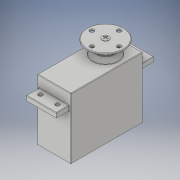
# Autodesk Inventor part: двигатель
Saved by Autodesk Inventor 2019 (Build 230136000, 136)
## iProperties
Created: 2019-09-05
Part Number: двигатель
Material: Типовые
Document SubType Name: Modeling
Designer: Iliga
Density: 1 g/cm^3
Appearance: По умолчанию
Author: Iliga
Autodesk Inventor part; units mm, degrees
sketch "Эскиз1" plane through (0, 0, 0) normal (0, 1, 0) x (-1, 0, 0)
  line L0 (-9.9, 21.15) -> (9.9, 21.15)
  line L1 (9.9, 21.15) -> (9.9, -21.15)
  line L2 (9.9, -21.15) -> (-9.9, -21.15)
  line L3 (-9.9, -21.15) -> (-9.9, 21.15)
  line L4 (-9.9, 21.15) -> (9.9, -21.15) construction
  line L5 (9.9, 21.15) -> (-9.9, -21.15) construction
  point P0 (0, 0)
  dimension "d0" = 19.8
  dimension "d1" = 42.3
  constraints: 12 end point, 2 midpoint, 2 parallel, 1 horizontal, 1 perpendicular
  measures "d0" distance of L1.end L2.end
  measures "d1" distance of L0.end L1.end
extrude "Выдавливание1" add sketch "Эскиз1" along normal blind 36.1
ref_plane "РабПлоскость1" through (0, 26.6, 0) normal (0, -1, 0) x (1, 0, 0)
sketch "Эскиз2" plane through (0, 26.6, 0) normal (0, -1, 0) x (1, 0, 0)
  line L0 (9.9, 21.15) -> (-9.9, 21.15) projected
  line L1 (-8.9, 28.75) -> (8.9, 28.75)
  line L2 (-9.9, -21.15) -> (9.9, -21.15) projected
  line L3 (-8.9, -28.75) -> (8.9, -28.75)
  line L4 (0, 28.75) -> (0, -28.75) construction
  line L5 (-9.9, 21.15) -> (9.9, 21.15)
  line L6 (9.9, -21.15) -> (9.9, 21.15) construction
  line L7 (-9.9, -21.15) -> (9.9, -21.15)
  line L8 (-8.9, 28.75) -> (-8.9, 21.15)
  line L9 (8.9, 28.75) -> (8.9, 21.15)
  line L10 (-8.9, -21.15) -> (-8.9, -28.75)
  line L11 (8.9, -21.15) -> (8.9, -28.75)
  line L12 (-9.9, 21.15) -> (-9.9, -21.15) projected
  point P0 (0, 0)
  point P1 (0, 0)
  dimension "d5" = 57.5
  dimension "d8" = 1
  constraints: 18 end point, 6 point on line, 4 perpendicular, 3 midpoint, 2 horizontal, 1 coincident, 1 collinear
  measures "d5" distance between parallel lines of L1 L3
  measures "d8" distance between parallel lines of L12 L10
extrude "Выдавливание2" add sketch "Эскиз2" against normal blind 3
sketch "Эскиз3" plane through (0, 36.1, 0) normal (0, 1, 0) x (1, 0, 0)
  circle A0 centre (0, 9.15) radius 7.5
  line L0 (9.9, 21.15) -> (-9.9, 21.15) construction
  line L1 (-9.9, 16.65) -> (9.9, 16.65) construction
  line L2 (-9.9, 21.15) -> (-9.9, -21.15) construction
  point P0 (0, 0)
  dimension "d9" = 15
  dimension "d53" = 4.5
  constraints: 2 end point, 2 vertical alignment, 1 centre point, 1 horizontal, 1 point on line, 1 tangent
  measures "d9" diameter of A0
  measures "d53" distance of L0.start L1.end
ref_plane "РабПлоскость2" through (0, 39.1, 0) normal (0, 1, 0) x (1, 0, 0)
sketch "Эскиз4" plane through (0, 39.1, 0) normal (0, 1, 0) x (1, 0, 0)
  circle A0 centre (0, 9.15) radius 7.5 construction
  circle A1 centre (0, 9.15) radius 5.75
  point P0 (0, 0)
  dimension "d11" = 11.5
  constraints: 1 centre point, 1 coincident
  measures "d11" diameter of A1
loft "Лофт1" add profiles "Эскиз3", "Эскиз4"
ref_plane "РабПлоскость3" through (0, 44.1, 0) normal (0, -1, 0) x (1, 0, 0)
sketch "Эскиз5" plane through (0, 44.1, 0) normal (0, -1, 0) x (1, 0, 0)
  circle A0 centre (0, -9.15) radius 5.75 construction
  circle A1 centre (0, -9.15) radius 10.75
  point P0 (0, 0)
  dimension "d17" = 21.5
  constraints: 1 centre point, 1 coincident
  measures "d17" diameter of A1
extrude "Выдавливание3" add sketch "Эскиз5" along normal blind 1
sketch "Эскиз6" plane through (0, 43.1, -9.15) normal (0, -1, 0) x (1, 0, 0)
  circle A0 centre (0, 0) radius 5.75 construction
  circle A1 centre (0, 0) radius 4.5
  circle A2 centre (0, 0) radius 3
  point P0 (0, 9.15)
  dimension "d20" = 9
  dimension "d21" = 6
  constraints: 2 centre point, 2 coincident
  measures "d20" diameter of A1
  measures "d21" diameter of A2
extrude "Выдавливание4" add sketch "Эскиз6" along normal blind 4 contours A2
extrude "Выдавливание5" add sketch "Эскиз6" along normal blind 3
sketch "Эскиз7" plane through (0, 44.1, -9.15) normal (0, 1, 0) x (1, 0, 0)
  circle A0 centre (0, 0) radius 8 construction
  circle A1 centre (0, -8) radius 1
  circle A2 centre (-8, 0) radius 1
  circle A3 centre (0, 8) radius 1
  circle A4 centre (8, 0) radius 1
  point P0 (0, -9.15)
  dimension "d26" = 16
  dimension "d27" = 2
  dimension "d28" = 2
  dimension "d29" = 2
  dimension "d30" = 2
  constraints: 5 centre point, 4 point on circle
  measures "d26" diameter of A0
  measures "d27" diameter of A1
  measures "d28" diameter of A2
  measures "d29" diameter of A3
  measures "d30" diameter of A4
ref_plane "РабПлоскость4" through (0, 44.1, -9.15) normal (1, 0, 0) x (0, 0, -1)
sketch "Эскиз8" plane through (0, 44.1, -9.15) normal (1, 0, 0) x (0, 0, -1)
  line L0 (-10.75, 0) -> (-10.75, 0)
  arc A0 (2, 0.2) -> (0, 0.6721) centre (0, -3.8) ccw
  line L1 (0, 0.6721) -> (0, 0)
  line L2 (2, 0) -> (0, 0)
  line L3 (10.75, 0) -> (-10.75, 0) projected
  line L4 (2, 0) -> (2, 0.2)
  point P0 (-9.15, -44.1)
  dimension "d31" = 2
  dimension "d32" = 0.2
  dimension "d33" = 3.8
  constraints: 9 end point, 2 point on circle, 2 vertical, 1 centre point, 1 midpoint, 1 perpendicular, 1 point on line, 1 vertical alignment
  measures "d31" distance of L1.end L2.start
  measures "d32" distance of L2.start L4.end
  measures "d33" distance of L1.end A0.centre
revolve "Вращение1" add sketch "Эскиз8" angle 360 about axis through (0, 44.7721, -9.15) along (0, -1, 0)
sketch "Эскиз9" plane through (0, 44.1, -9.15) normal (0, 1, 0) x (1, 0, 0)
  line L0 (-0.25, -0.25) -> (-1.25, -0.25)
  line L1 (-1.25, -0.25) -> (-1.25, 0.25)
  line L2 (-1.25, 0.25) -> (-0.25, 0.25)
  line L3 (-0.25, 0.25) -> (-0.25, 1.25)
  line L4 (-0.25, 1.25) -> (0.25, 1.25)
  line L5 (0.25, 1.25) -> (0.25, 0.25)
  line L6 (0.25, 0.25) -> (1.25, 0.25)
  line L7 (1.25, 0.25) -> (1.25, -0.25)
  line L8 (1.25, -0.25) -> (0.25, -0.25)
  line L9 (0.25, -0.25) -> (0.25, -1.25)
  line L10 (0.25, -1.25) -> (-0.25, -1.25)
  line L11 (-0.25, -1.25) -> (-0.25, -0.25)
  line L12 (0.25, -0.25) -> (-0.25, 0.25) construction
  line L13 (0.25, 0.25) -> (-0.25, -0.25) construction
  line L14 (9.9, -30.3) -> (-9.9, -30.3) projected
  line L15 (-9.9, -30.3) -> (-9.9, 12) projected
  line L16 (-9.9, 12) -> (9.9, 12) projected
  line L17 (9.9, 12) -> (9.9, -30.3) projected
  circle A0 centre (0, 0) radius 10.75 projected
  point P0 (0, -9.15)
  point P1 (0.25, 0.75)
  point P2 (0.25, -0.75)
  point P3 (0, 0)
  point P4 (0, 0)
  dimension "d35" = 0.5
  dimension "d36" = 0.5
  dimension "d37" = 1
  constraints: 28 end point, 7 perpendicular, 4 midpoint, 3 equal length, 3 point on line, 2 horizontal alignment, 2 parallel, 1 coincident, 1 vertical, 1 vertical alignment
  measures "d35" distance between parallel lines of L0 L2
  measures "d36" distance between parallel lines of L3 L5
  measures "d37" distance of L9.end L8.end
extrude "Выдавливание6" cut sketch "Эскиз9" along normal up to surface contours L0 L1 L2 L3 L4 L5 L6 L7 L8 L9 L10 L11
extrude "Выдавливание7" cut sketch "Эскиз7" against normal up to surface (1 mm away)
sketch "Эскиз10" plane through (0, 29.6, 0) normal (0, 1, 0) x (1, 0, 0)
  circle A0 centre (-5, -24.15) radius 1
  circle A1 centre (5, -24.15) radius 1
  line L0 (5, -24.15) -> (-5, -24.15) construction
  line L1 (-8.9, -28.75) -> (8.9, -28.75) projected
  line L2 (8.9, -21.15) -> (-8.9, -21.15) projected
  point P0 (0, 0)
  point P1 (0, -24.15)
  dimension "d42" = 10
  dimension "d43" = 2
  dimension "d44" = 2
  dimension "d54" = 3
  constraints: 2 centre point, 2 end point, 1 horizontal, 1 midpoint, 1 vertical alignment
  measures "d42" distance of L0.end L0.start
  measures "d43" diameter of A0
  measures "d44" diameter of A1
  measures "d54" distance from line of L2 point (0, -24.15)
extrude "Выдавливание8" cut sketch "Эскиз10" against normal up to surface (3 mm away)
pattern_linear "Прямоуг.массив1" count 2 spacing 48.3 along (0, 0, -1) of "Выдавливание8"
fillet "Сопряжение1" radius 0.3 58 edges at (8.9, 29.6, 24.95) (0, 29.6, 28.75) (4, 29.6, 24.15) (-6, 29.6, 24.15) (-8.9, 29.6, 24.95) (0, 26.6, 28.75) (-8.9, 28.1, 28.75) (-8.9, 26.6, 24.95) (-6, 26.6, 24.15) (4, 26.6, 24.15) (8.9, 26.6, 24.95) (8.9, 29.6, -24.95) (8.9, 26.6, -24.95) (8.9, 28.1, -28.75) (0, 29.6, -28.75) (0, 26.6, -28.75) (4, 29.6, -24.15) (-6, 29.6, -24.15) (-8.9, 29.6, -24.95) (-8.9, 28.1, -28.75) (0, 29.6, -21.15) (0, 26.6, -21.15) (4, 26.6, -24.15) (-6, 26.6, -24.15) (8.9, 28.1, -21.15) (-8.9, 28.1, -21.15) (-8.9, 26.6, -24.95) (-8.9, 28.1, 21.15) (0, 29.6, 21.15) (8.9, 28.1, 21.15) (0, 26.6, 21.15) (9.9, 36.1, 0) (0, 36.1, 21.15) (-9.9, 36.1, 0) (0, 36.1, -21.15) (9.9, 18.05, -21.15) (9.9, 18.05, 21.15) (-9.9, 18.05, 21.15) (-9.9, 18.05, -21.15) (-9.9, 0, 0) (0, 0, -21.15) (9.9, 0, 0) (0, 0, 21.15) (-7.5, 36.1, -9.15) (-3, 39.1, -9.15) (-5.75, 39.1, -9.15) (-4.5, 40.1, -9.15) (-4.5, 43.1, -9.15) (-10.75, 43.1, -9.15) (-10.75, 44.1, -9.15) (-1, 44.1, -17.15) (-9, 44.1, -9.15) (-1, 44.1, -1.15) (7, 44.1, -9.15) (-1, 43.1, -17.15) (7, 43.1, -9.15) (-1, 43.1, -1.15) (-9, 43.1, -9.15)
